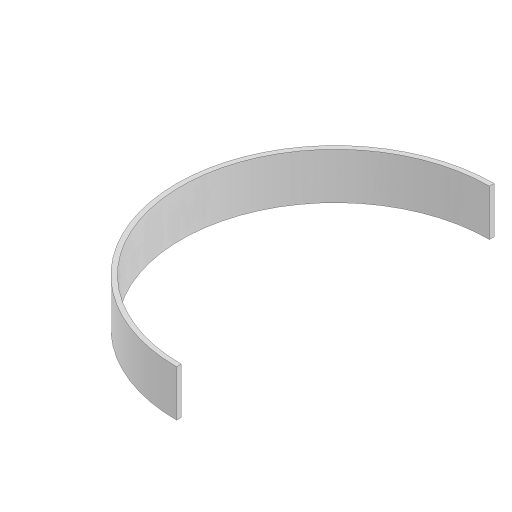
# Autodesk Inventor part: R10_CM_CIRCULO
Saved by Autodesk Inventor 2024.2 (Build 282272000, 272)
## iProperties
Created: 2024-10-01
Part Number: R10_CM_CIRCULO
Material: Generic
Document SubType Name: Modeling
Designer: jrcer
Density: 1 g/cm^3
Appearance: Default
Author: jrcer
Autodesk Inventor part; units mm, degrees
ref_plane "YZ Plane" through (0, 0, 0) normal (1, 0, 0) x (0, 1, 0)
ref_plane "XZ Plane" through (0, 0, 0) normal (0, 1, 0) x (-1, 0, 0)
ref_plane "XY Plane" through (0, 0, 0) normal (0, 0, 1) x (1, 0, 0)
sketch "Sketch1" plane through (0, 0, 0) normal (0, 1, 0) x (-1, 0, 0)
  circle A0 centre (0, 0) radius 100
  circle A1 centre (0, 0) radius 103
  line L0 (0, -100) -> (0, -103)
  line L1 (0, 100) -> (0, 103)
  point P0 (0, 101.5)
  dimension "d0" = 200
  dimension "d1" = 206
  constraints: 4 end point, 4 point on circle, 2 centre point, 2 coincident, 2 vertical, 2 vertical alignment, 1 midpoint
  measures "d0" diameter of A0
  measures "d1" diameter of A1
extrude "Extrusion1" add sketch "Sketch1" along normal blind 30 contours A0 L1 A1 L0 picked at (101.4211, -8.8323)
body "Solid1"
